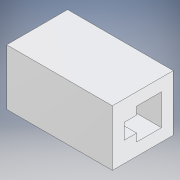
# Autodesk Inventor part: Ethernet Port
Saved by Autodesk Inventor 2017 SP1 (Build 210196100, 196)
## iProperties
Created: 2017-09-20
Part Number: Ethernet Port
Material: ABS Plastic
Document SubType Name: Modeling
Designer: Zach
Density: 1.06 g/cm^3
Appearance: CR White
Author: Zach
Autodesk Inventor part; units mm, degrees
ref_plane "YZ Plane" through (0, 0, 0) normal (1, 0, 0) x (0, 1, 0)
ref_plane "XZ Plane" through (0, 0, 0) normal (0, 1, 0) x (-1, 0, 0)
ref_plane "XY Plane" through (0, 0, 0) normal (0, 0, 1) x (1, 0, 0)
sketch "Sketch1" plane through (0, 0, 0) normal (0, 0, 1) x (1, 0, 0)
  line L0 (0, 0) -> (43.18, 0)
  line L1 (43.18, 0) -> (43.18, 22.86)
  line L2 (43.18, 22.86) -> (0, 22.86)
  line L3 (0, 22.86) -> (0, 0)
  dimension "d0" = 43.18
  dimension "d1" = 22.86
  constraints: 8 end point, 2 parallel, 1 horizontal, 1 perpendicular
  measures "d0" distance of L2.end L1.end
  measures "d1" distance of L1.end L0.end
extrude "Extrusion1" add sketch "Sketch1" along normal blind 24.892
sketch "Sketch2" plane through (43.18, 0, 0) normal (1, 0, 0) x (0, 0, -1)
  line L0 (-4.826, 5.08) -> (-14.986, 5.08)
  line L1 (-14.986, 5.08) -> (-14.986, 17.78)
  line L2 (-14.986, 17.78) -> (-4.826, 17.78)
  line L3 (-4.826, 17.78) -> (-4.826, 5.08)
  line L4 (-24.892, 0) -> (-24.892, 22.86) construction
  line L5 (-14.986, 8.255) -> (-20.066, 8.255)
  line L6 (-20.066, 8.255) -> (-20.066, 14.605)
  line L7 (-20.066, 14.605) -> (-14.986, 14.605)
  line L8 (-14.986, 14.605) -> (-14.986, 8.255)
  line L9 (-20.066, 17.78) -> (-4.826, 17.78)
  line L10 (0, 22.86) -> (-24.892, 22.86) construction
  point P0 (0, 0)
  point P1 (-14.986, 11.43)
  point P2 (-24.892, 11.43)
  point P3 (-20.066, 11.43)
  point P4 (-12.446, 17.78)
  point P5 (-12.446, 22.86)
  dimension "d4" = 10.16
  dimension "d5" = 12.7
  dimension "d6" = 5.08
  dimension "d7" = 6.35
  constraints: 18 end point, 6 midpoint, 4 parallel, 3 horizontal, 2 horizontal alignment, 2 perpendicular, 2 vertical alignment, 1 point on line
  measures "d4" distance of L1.end L2.end
  measures "d5" distance of L0.end L1.end
  measures "d6" distance of L6.end L7.end
  measures "d7" distance of L5.end L6.end
extrude "Extrusion2" cut sketch "Sketch2" against normal blind 12.7
sketch "Sketch3" plane through (0, 0, 0) normal (-1, 0, 0) x (0, 0, 1)
  line L0 (14.986, 14.605) -> (14.986, 17.78) projected
  line L1 (20.066, 14.605) -> (14.986, 14.605) projected
  line L2 (20.066, 8.255) -> (20.066, 14.605) projected
  line L3 (14.986, 8.255) -> (20.066, 8.255) projected
  line L4 (4.826, 5.08) -> (14.986, 5.08) projected
  line L5 (4.826, 17.78) -> (4.826, 5.08) projected
  line L6 (14.986, 17.78) -> (4.826, 17.78) projected
  line L7 (14.986, 5.08) -> (14.986, 8.255) projected
  point P0 (0, 0)
extrude "Extrusion3" cut sketch "Sketch3" against normal blind 12.7
body "Solid1"
